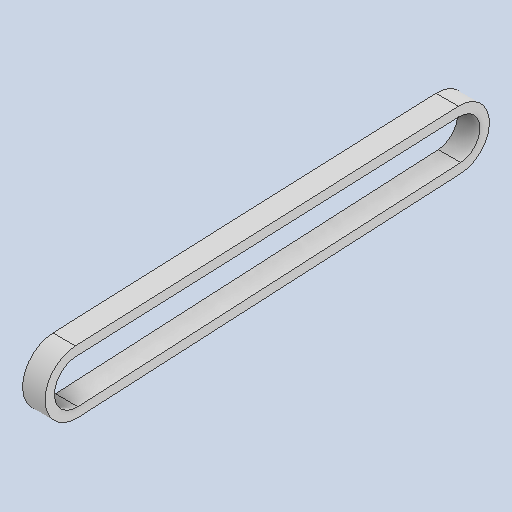
# Autodesk Inventor part: drivetimingbelt77mm
Saved by Autodesk Inventor 2023 (Build 270158000, 158)
## iProperties
Created: 2022-09-10
Part Number: drivetimingbelt77mm
Material: Generic
Document SubType Name: Modeling
Designer: deli
Density: 1 g/cm^3
Appearance: Default
Author: deli
Autodesk Inventor part; units mm, degrees
ref_plane "YZ Plane" through (0, 0, 0) normal (1, 0, 0) x (0, 1, 0)
ref_plane "XZ Plane" through (0, 0, 0) normal (0, 1, 0) x (-1, 0, 0)
ref_plane "XY Plane" through (0, 0, 0) normal (0, 0, 1) x (1, 0, 0)
sketch "Sketch1" plane through (0, 0, 0) normal (1, 0, 0) x (0, 1, 0)
  circle A0 centre (36.1899, -46.7573) radius 7 construction
  circle A1 centre (36.1899, -4.1748) radius 7 construction
  circle A2 centre (43.4399, 149.5339) radius 2 construction
  circle A3 centre (43.4399, -200.4661) radius 2 construction
  arc A4 (31.5196, -201.0901) -> (55.366, -199.9654) centre (43.4399, -200.4661) ccw
  arc A5 (48.911, -46.2232) -> (23.4749, -47.423) centre (36.1899, -46.7573) ccw
  line L0 (31.5196, -201.0901) -> (23.4749, -47.423)
  line L1 (55.366, -199.9654) -> (48.911, -46.2232)
  line L2 (45.1144, -46.3826) -> (51.5693, -200.1248)
  arc A6 (35.3144, -200.8915) -> (51.5693, -200.1248) centre (43.4399, -200.4661) ccw
  line L3 (35.3144, -200.8915) -> (27.2697, -47.2243)
  arc A7 (45.1144, -46.3826) -> (27.2697, -47.2243) centre (36.1899, -46.7573) ccw
  dimension "d0" = 23.8732
  dimension "d2" = 25.4648
  dimension "d4" = 3.8
  constraints: 8 end point, 8 point on circle, 4 centre point, 4 tangent, 2 coincident, 3 other
  measures "d0" diameter of A4
  measures "d2" diameter of A5
  measures "d4" distance between parallel lines of L1 L2
extrude "Extrusion1" add sketch "Sketch1" along normal blind 9
body "Solid1"
